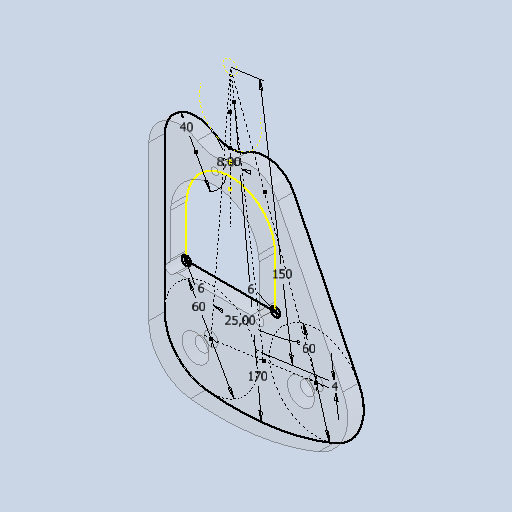
# Autodesk Inventor part: DPM_Counterweight_Fixation
Saved by Autodesk Inventor 2022 (Build 260153000, 153)
## iProperties
Created: 2022-10-25
Part Number: DPM_Counterweight_Fixation
Material: PMMA-Kunststoff
Document SubType Name: Modeling
Designer: alexw
Density: 1.188 g/cm^3
Appearance: Polycarbonat - klar
Mass: 144.79 g
Surface Area: 318.681 cm^2
Volume: 121.877 cm^3
COG_Offset: 4,000 mm
Author: alexw
Autodesk Inventor part; units mm, degrees
ref_plane "YZ Plane" through (0, 0, 0) normal (1, 0, 0) x (0, 1, 0)
ref_plane "XZ Plane" through (0, 0, 0) normal (0, 1, 0) x (-1, 0, 0)
ref_plane "XY Plane" through (0, 0, 0) normal (0, 0, 1) x (1, 0, 0)
sketch "Skizze1" plane through (0, 0, 0) normal (0, 0, 1) x (1, 0, 0)
  arc A0 (28.1111, -17.5491) -> (-28.1111, -17.5491) centre (0, -21.25) ccw projected
  arc A1 (-19.0016, 48.9902) -> (19.0016, 48.9902) centre (0, 42.75) ccw construction
  line L0 (-28.1111, -17.5491) -> (-28.5983, -21.25) projected
  line L1 (-28.5983, -21.25) -> (-28.5983, -53.75) projected
  line L2 (28.5983, -21.25) -> (28.1111, -17.5491) projected
  line L3 (28.5983, -53.75) -> (28.5983, -21.25) projected
  line L4 (1.5, -53.75) -> (28.5983, -53.75) construction
  line L5 (-28.5983, -53.75) -> (-1.5, -53.75) construction
  line L6 (-28.5983, -53.75) -> (28.5983, -53.75)
  circle A2 centre (0, 67.75) radius 4.5 construction
  line L7 (0, 67.75) -> (20.876, -80.7902) construction
  line L8 (0, 67.75) -> (0, -21.25) construction
  arc A3 (-11.188, 26.1721) -> (11.188, 26.1721) centre (0, 42.75) ccw
  arc A4 (-11.188, 26.1721) -> (-42.3761, 9.5941) centre (-22.3761, 9.5941) ccw
  arc A5 (40.3275, 18.4115) -> (11.188, 26.1721) centre (22.3761, 9.5941) ccw
  line L9 (-42.3761, 9.5941) -> (-42.3761, -89.5028)
  line L10 (40.3275, 18.4115) -> (82.1686, -66.7738)
  circle A6 centre (0, 14.8537) radius 1.621 construction
  circle A7 centre (-12.3761, -89.5028) radius 30 construction
  arc A8 (-15.5716, -119.3321) -> (66.5352, -107.7927) centre (2.5367, 49.7007) ccw
  circle A9 centre (55.2414, -79.9998) radius 30 construction
  arc A10 (-42.3761, -89.5028) -> (-15.5716, -119.3321) centre (-12.3761, -89.5028) ccw
  arc A11 (66.5352, -107.7927) -> (82.1686, -66.7738) centre (55.2414, -79.9998) ccw
  line L11 (-12.3761, -89.5028) -> (55.2414, -79.9998) construction
  line L12 (0, 67.75) -> (-12.3761, -89.5028) construction
  line L13 (0, 67.75) -> (55.2414, -79.9998) construction
  circle A12 centre (-28.5983, -53.75) radius 3
  circle A13 centre (28.5983, -53.75) radius 3
  point P0 (0, 0)
  point P1 (0, 22.75)
  point P2 (28.5983, -50.75)
  point P3 (25.5983, -53.75)
  point P4 (-25.5983, -53.75)
  point P5 (-28.5983, -50.75)
  point P6 (21.4327, -84.7513)
  dimension "d0" = 150
  dimension "d1" = 8
  dimension "d2" = 60
  dimension "d3" = 60
  dimension "d4" = 40
  dimension "d5" = 25
  dimension "d6" = 170
  dimension "d7" = 6
  dimension "d8" = 6
  dimension "COG_Offset" = 4
  constraints: 18 point on circle, 16 end point, 11 tangent, 10 centre point, 6 coincident, 2 equal radius, 1 concentric, 1 horizontal, 1 midpoint, 1 parallel, 1 perpendicular, 1 point on line, 1 vertical
  measures "d0" distance of L7.end L7.start
  measures "d1" angle of L7 L8
  measures "d2" diameter of A7
  measures "d3" diameter of A9
  measures "d4" diameter of A4
  measures "d5" angle of L13 L12
  measures "d6" radius of A8
  measures "d7" diameter of A12
  measures "d8" diameter of A13
  measures "COG_Offset" distance from line of L7.end L11
extrude "Extrusion1" add sketch "Skizze1" along normal blind 10
fillet "Rundung1" radius 3 4 edges at (-28.5983, -50.75, 5) (-25.5983, -53.75, 5) (28.5983, -50.75, 5) (25.5983, -53.75, 5)
hole "Bohrung1" at (0, 14.8537, 0) direction (0, 0, 1) diameter 4.5 end through all clearance for "Innensechskant-Senkkopfschraube DIN EN ISO 10642" size "M4" standard "DIN"
hole "Bohrung2" at (-12.3761, -89.5028, 0) at (55.2414, -79.9998, 0) direction (0, 0, 1) diameter 9 end through all clearance for "Innensechskant-Senkkopfschraube DIN EN ISO 10642" size "M8" standard "DIN"
thicken "Verdickung1" operation add thickness 0.1 both sides no extend neighbours yes toward (1, 0, 0) faces at (-28.5983, -39.4526, 3.3333) (-28.4359, -20.0164, 3.3333) (27.1625, -13.1181, 6.6667) (28.2735, -18.7827, 3.3333) (28.5983, -30.3513, 3.3333) (7.8007, -53.75, 3.3333)
sketch "Skizze2" plane through (0, 0, 10) normal (0, 0, 1) x (1, 0, 0)
  point P0 (0, 0)
  point P1 (-12.3761, -89.5028)
  point P2 (55.2414, -79.9998)
hole "Bohrung3" at (-12.3761, -89.5028, 10) at (55.2414, -79.9998, 10) direction (0, 0, -1) diameter 9 end through all countersink diameter 17.3 countersink angle 90 clearance for "Flachkopfsenkschraube DIN EN ISO 2009" size "M8" standard "DIN"
